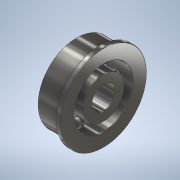
# Autodesk Inventor part: F606ZZFlanged
Saved by Autodesk Inventor 2021 (Build 250183000, 183)
## iProperties
Created: 2019-09-20
Part Number: F606ZZFlanged
Material: Generic
Document SubType Name: Modeling
Designer: xyz-150G
Density: 1 g/cm^3
Appearance: Steel - Polished
Mass: 1.81571 g
Surface Area: 20.7306 cm^2
Volume: 1.81571 cm^3
Author: xyz-150G
Autodesk Inventor part; units mm, degrees
ref_plane "YZ Plane" through (0, 0, 0) normal (1, 0, 0) x (0, 1, 0)
ref_plane "XZ Plane" through (0, 0, 0) normal (0, 1, 0) x (-1, 0, 0)
ref_plane "XY Plane" through (0, 0, 0) normal (0, 0, 1) x (1, 0, 0)
sketch "Sketch2" plane through (0, 0, 0) normal (0, 0, 1) x (1, 0, 0)
  line L0 (-5.9, 2.5) -> (-0.1, 2.5)
  line L1 (0, 2.6) -> (0, 4.4667)
  line L2 (-0.1, 4.5667) -> (-5.9, 4.5667)
  line L3 (-6, 4.4667) -> (-6, 2.6)
  line L4 (-5.9, 8.5) -> (-1.0707, 8.5)
  line L5 (-0.1, 6.4333) -> (-5.9, 6.4333)
  line L6 (-6, 6.5333) -> (-6, 8.4)
  line L7 (-1, 8.5) -> (-1, 8.5707) construction
  line L8 (-0.9, 9.5) -> (-0.1, 9.5)
  line L9 (-2.3, 0) -> (0, 0)
  line L10 (-6, 4.5667) -> (-6, 6.4333) construction
  line L11 (0, 0) -> (0, 2.5) construction
  line L12 (0, 6.5333) -> (0, 9.4)
  line L13 (-1.0707, 8.5) -> (-1, 8.4293)
  line L14 (-1.0707, 8.5) -> (-0.9707, 8.5) construction
  line L15 (-1, 8.4293) -> (-0.9293, 8.5)
  line L16 (-0.9293, 8.5) -> (-1, 8.5707)
  line L17 (-0.9646, 8.4646) -> (-1, 8.5) construction
  line L18 (-1, 8.5707) -> (-1, 9.4)
  line L19 (-1.0707, 8.5) -> (-1, 8.5) construction
  line L20 (-6, 8.4) -> (-5.9, 8.5)
  line L21 (-6, 6.5333) -> (-5.9, 6.4333)
  line L22 (-5.9, 4.5667) -> (-6, 4.4667)
  line L23 (-6, 2.6) -> (-5.9, 2.5)
  line L24 (-0.1, 2.5) -> (0, 2.6)
  line L25 (0, 4.4667) -> (-0.1, 4.5667)
  line L26 (-0.1, 6.4333) -> (0, 6.5333)
  line L27 (0, 9.4) -> (-0.1, 9.5)
  line L28 (-0.9, 9.5) -> (-1, 9.4)
  point P0 (0, 0)
  point P1 (-6, 2.5)
  point P2 (0, 4.5667)
  point P3 (-6, 8.5)
  point P4 (0, 6.4333)
  point P5 (-1, 9.5)
  point P6 (0, 9.5)
  dimension "d" = 5
  dimension "D" = 17
  dimension "C2" = 1
  dimension "d5" = 45
  dimension "d6" = 0.1
  dimension "D2" = 19
  dimension "d8" = 0.1
  dimension "d9" = 0.1
  dimension "d10" = 0.1
  dimension "d11" = 0.1
  dimension "d12" = 0.1
  dimension "d13" = 0.1
  dimension "d14" = 0.1
  dimension "d15" = 0.1
  dimension "d16" = 0.1
  dimension "d17" = 0.1
  dimension "d18" = 0.1
  dimension "d19" = 0.1
  dimension "d20" = 0.1
  dimension "d21" = 0.1
  dimension "d22" = 0.1
  dimension "d23" = 0.1
  dimension "d24" = 0.1
  dimension "d25" = 0.1
  dimension "bd" = 1.8667
  dimension "B1" = 6
  constraints: 58 end point, 20 point on line, 6 parallel, 5 horizontal, 4 equal length, 4 perpendicular, 3 vertical, 1 coincident, 1 collinear, 1 midpoint
  measures "d" diameter of L0 L9
  measures "D" diameter of L4 L9
  measures "C2" distance of point (-1, 9.5) point (0, 9.5)
  measures "d5" angle of L13 L14
  measures "d6" distance of L13.end L15.end
  measures "D2" diameter of L8 L9
  measures "d8" distance of L6.end point (-6, 8.5)
  measures "d9" distance of L4.start point (-6, 8.5)
  measures "d10" distance of L6.start L10.end
  measures "d11" distance of L5.end L10.end
  measures "d12" distance of L2.end L10.start
  measures "d13" distance of L3.start L10.start
  measures "d14" distance of L3.end point (-6, 2.5)
  measures "d15" distance of L0.start point (-6, 2.5)
  measures "d16" distance of L0.end L11.end
  measures "d17" distance of L1.start L11.end
  measures "d18" distance of L1.end point (0, 4.567)
  measures "d19" distance of L2.start point (0, 4.567)
  measures "d20" distance of L5.start point (0, 6.433)
  measures "d21" distance of L12.start point (0, 6.433)
  measures "d22" distance of L12.end point (0, 9.5)
  measures "d23" distance of L8.end point (0, 9.5)
  measures "d24" distance of L8.start point (-1, 9.5)
  measures "d25" distance of L18.end point (-1, 9.5)
  measures "bd" distance between parallel lines of L2 L5
  measures "B1" distance between parallel lines of L12 L6
revolve "Revolution1" add sketch "Sketch2" angle 360 about axis through (-2.3, 0, 0) along (1, 0, 0)
sketch "Sketch3" plane through (0, 0, 0) normal (0, 0, 1) x (1, 0, 0)
  line L0 (-0.1, 6.4333) -> (-5.9, 6.4333) construction
  line L1 (-5.9, 4.5667) -> (-0.1, 4.5667) construction
  line L2 (-3, 6.4333) -> (-3, 4.5667)
  arc A0 (-3, 4.38) -> (-3, 6.62) centre (-3, 5.5) ccw construction
  line L3 (-3, 6.4333) -> (-3, 6.62)
  line L4 (-3, 4.5667) -> (-3, 4.38)
  arc A1 (-3.6191, 4.5667) -> (-3, 4.38) centre (-3, 5.5) ccw
  arc A2 (-3, 6.62) -> (-3.6191, 4.5667) centre (-3, 5.5) ccw
  point P0 (0, 0)
  dimension "d28" = 2.24
  constraints: 6 end point, 6 point on circle, 3 centre point, 3 midpoint, 2 point on line, 1 perpendicular, 1 vertical
  measures "d28" diameter of A0
revolve "Revolution2" add sketch "Sketch3" angle 360 about axis through (-3, 6.4333, 0) along (0, -1, 0)
pattern_circular "Circular Pattern1" count 6 over 360 about axis through (-10, 0, 0) along (1, 0, 0) of "Revolution2"
equation "\"d6\" = 0.1 * C2"
equation "\"d8\" = 0.1 * C2"
equation "\"d9\" = d8"
equation "\"d10\" = d8"
equation "\"d11\" = d10"
equation "\"d12\" = d8"
equation "\"d13\" = d12"
equation "\"d14\" = d8"
equation "\"d15\" = d14"
equation "\"d16\" = d8"
equation "\"d17\" = d16"
equation "\"d18\" = d8"
equation "\"d19\" = d18"
equation "\"d20\" = d8"
equation "\"d21\" = d20"
equation "\"d22\" = d8"
equation "\"d23\" = d22"
equation "\"d24\" = d8"
equation "\"d25\" = d24"
equation "\"d28\" = 1.2 * bd"
body "Solid1"
